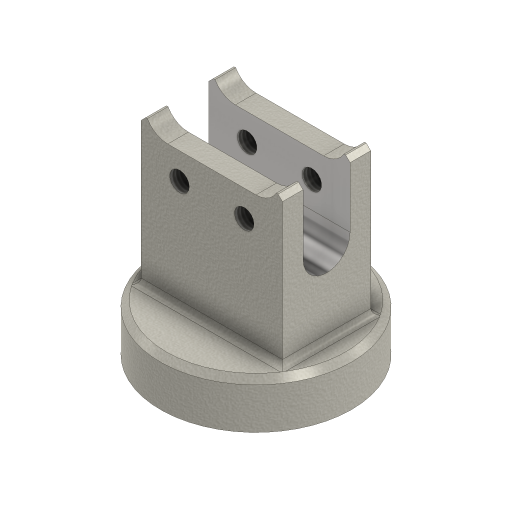
# Autodesk Inventor part: Part014. Pivoting support
Saved by Autodesk Inventor 2023.2 (Build 272271030, 271C)
## iProperties
Created: 2023-09-13
Part Number: Part014. Pivoting support
Material: Steel, Cast
Document SubType Name: Modeling
Designer: User
Mass: 711.293 g
Surface Area: 231.914 cm^2
Volume: 90.6105 cm^3
Density: 7.85 g/cm^3
Appearance: Steel - Cast
Author: User
Autodesk Inventor part; units mm, degrees
ref_plane "YZ Plane" through (0, 0, 0) normal (1, 0, 0) x (0, 1, 0)
ref_plane "XZ Plane" through (0, 0, 0) normal (0, 1, 0) x (-1, 0, 0)
ref_plane "XY Plane" through (0, 0, 0) normal (0, 0, 1) x (1, 0, 0)
sketch "Sketch1" plane through (0, 0, 0) normal (0, 0, 1) x (1, 0, 0)
  line L0 (0, 0) -> (0, 24)
  line L1 (0, 24) -> (32.5, 24)
  line L2 (32.5, 24) -> (32.5, 8)
  line L3 (32.5, 8) -> (27.5, 8)
  line L4 (27.5, 8) -> (27.5, 12)
  line L5 (27.5, 12) -> (22.5, 12)
  line L6 (22.5, 12) -> (22.5, 8)
  line L7 (22.5, 8) -> (18, 8)
  line L8 (18, 8) -> (18, 0)
  line L9 (18, 0) -> (0, 0)
  point P0 (25, 12)
  dimension "d0" = 65
  dimension "d1" = 36
  dimension "d2" = 8
  dimension "d3" = 16
  dimension "d4" = 45
  dimension "d5" = 55
  dimension "d6" = 4
  constraints: 20 end point, 8 perpendicular, 2 point on line, 1 midpoint, 1 vertical
  measures "d0" diameter of L2 L0
  measures "d1" diameter of L8 L0
  measures "d2" distance between parallel lines of L9 L7
  measures "d3" distance between parallel lines of L7 L1
  measures "d4" diameter of L6 L0
  measures "d5" diameter of L4 L0
  measures "d6" distance from line of L3 point (25, 12)
revolve "Revolution1" add sketch "Sketch1" angle 360 about axis through (0, 0, 0) along (0, 1, 0)
chamfer "Chamfer1" distance 2 angle 45 1 edges at (-32.5, 24, 0)
chamfer "Chamfer2" distance 1.5 angle 45 1 edges at (-18, 0, 0)
sketch "Sketch2" plane through (0, 0, 0) normal (0, 0, 1) x (1, 0, 0)
  line L0 (-30.5, 24) -> (30.5, 24) projected
  line L1 (24, 24) -> (-24, 24)
  line L2 (-24, 24) -> (-24, 74)
  line L3 (-24, 74) -> (-21.9282, 74)
  line L4 (24, 74) -> (24, 24)
  line L5 (15, 70) -> (-15, 70)
  arc A0 (-21.9282, 74) -> (-15, 70) centre (-15, 78) ccw
  line L6 (0, -19.6) -> (0, 117.6) construction
  line L7 (32.5, 8) -> (-32.5, 8) construction
  line L8 (16.5, 0) -> (-16.5, 0) construction
  arc A1 (15, 70) -> (21.9282, 74) centre (15, 78) ccw
  line L9 (21.9282, 74) -> (24, 74)
  line L10 (-21.9282, 74) -> (21.9282, 74) construction
  point P0 (0, 0)
  point P1 (0, 24)
  point P2 (0, 24)
  point P3 (1.0921, 70)
  dimension "d14" = 48
  dimension "d16" = 8
  dimension "d18" = 74
  dimension "d19" = 62
  dimension "d20" = 30
  constraints: 14 end point, 4 parallel, 4 point on circle, 3 symmetric about line, 2 centre point, 2 horizontal, 2 midpoint, 2 point on line, 1 coincident, 1 perpendicular, 1 tangent, 1 other
  measures "d14" distance between parallel lines of L4 L2
  measures "d16" radius of A0
  measures "d18" distance between parallel lines of L8 L3
  measures "d19" distance from line of L7 point (1.092, 70)
  measures "d20" distance of A1.centre A0.centre
extrude "Extrusion1" add sketch "Sketch2" along normal mid plane 30
chamfer "Chamfer3" distance 1.5 angle 45 2 edges at (24, 74, 0) (-24, 74, 0)
sketch "Sketch3" plane through (24, 24, 15) normal (1, 0, 0) x (0, 0, -1)
  line L0 (30, 50) -> (0, 50) construction
  line L1 (7, 50) -> (7, 28)
  arc A0 (7, 28) -> (23, 28) centre (15, 28) ccw
  line L2 (23, 28) -> (23, 50)
  line L3 (23, 50) -> (7, 50)
  line L4 (47.5, -16) -> (-17.5, -16) projected
  point P0 (15, -24)
  dimension "d26" = 44
  dimension "d27" = 8
  constraints: 6 end point, 2 parallel, 2 point on circle, 2 point on line, 1 centre point, 1 horizontal, 1 tangent, 1 vertical, 1 vertical alignment
  measures "d26" distance from line of L4 A0.centre
  measures "d27" radius of A0
extrude "Extrusion2" cut sketch "Sketch3" against normal through all
sketch "Sketch4" plane through (0, 0, 0) normal (0, -1, 0) x (1, 0, 0)
  circle A0 centre (0, 0) radius 16.5 projected
  point P0 (0, 0)
  constraints: 1 coincident
hole "Hole1" at (0, 0, 0) direction (0, 1, 0) diameter 22 depth 35 tip angle 118
sketch "Sketch5" plane through (0, 0, 15) normal (0, 0, 1) x (1, 0, 0)
  line L0 (-11, 61) -> (11, 61) construction
  line L1 (32.5, 8) -> (-32.5, 8) projected
  point P0 (0, 0)
  point P1 (0, 61)
  dimension "d37" = 22
  dimension "d38" = 53
  constraints: 2 end point, 1 horizontal, 1 midpoint, 1 vertical alignment
  measures "d37" distance of L0.end L0.start
  measures "d38" distance from line of L1 L0.end
hole "Hole2" at (-11, 61, 15) at (11, 61, 15) direction (0, 0, -1) diameter 6.647 end through all thread size "M8x1.25" class "6H" standard "ISO Metric profile"
fillet "Fillet1" radius 2 4 edges at (0, 24, 15) (24, 24, 0) (-24, 24, 0) (0, 24, -15)
body "Solid1"
